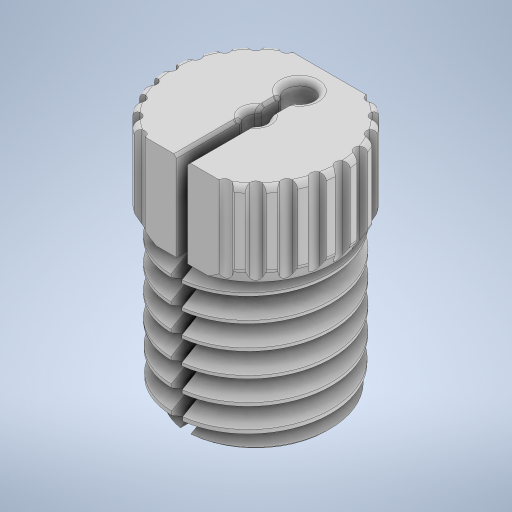
# Autodesk Inventor part: Ferula FOV5
Saved by Autodesk Inventor 2024.2 (Build 282272000, 272)
## iProperties
Created: 2025-08-06
Part Number: Ferula FOV5
Material: Generic
Document SubType Name: Modeling
Designer: ja.restrepo1
Density: 1 g/cm^3
Appearance: Default
Author: ja.restrepo1
Autodesk Inventor part; units mm, degrees
ref_plane "YZ Plane" through (0, 0, 0) normal (1, 0, 0) x (0, 1, 0)
ref_plane "XZ Plane" through (0, 0, 0) normal (0, 1, 0) x (-1, 0, 0)
ref_plane "XY Plane" through (0, 0, 0) normal (0, 0, 1) x (1, 0, 0)
sketch "Sketch1" plane through (0, 0, 0) normal (1, 0, 0) x (0, 0, -1)
  line L0 (-0.725, 5.6) -> (-0.725, 10.6)
  line L1 (-0.725, 10.6) -> (-5.825, 10.6)
  line L2 (-2.7455, -0.9529) -> (-2.1722, 5.6)
  line L3 (-2.1722, 5.6) -> (-0.725, 5.6)
  line L4 (-5.825, 3.6) -> (-5.756, -0.353)
  line L5 (-5.1455, -0.9529) -> (-2.7455, -0.9529)
  line L6 (-5.825, 10.6) -> (-5.825, 3.6)
  line L7 (0, -3.2635) -> (0, 12.9106) projected
  line L8 (-5.1455, -0.9529) -> (-5.756, -0.353)
  point P0 (0, 0)
  point P1 (-5.7455, -0.9529)
  point P2 (0, 0)
  dimension "d1" = 5
  dimension "d4" = 3
  dimension "d8" = 7
  dimension "d11" = 0.725
  dimension "d12" = 5.1
  dimension "d13" = 179
  dimension "d41" = 5.825
  dimension "d65" = 0.6
  dimension "d66" = 0.6
  dimension "d67" = 11.5529
  dimension "d98" = 5.6
  dimension "d100" = 95
  dimension "d111" = 1.4472
  constraints: 17 end point, 2 coincident, 2 perpendicular, 2 point on line, 1 horizontal, 1 parallel, 1 vertical
  measures "d1" distance of L3.end L0.end
  measures "d4" distance of point (-5.746, -0.953) L5.end
  measures "d8" distance of L6.start L4.start
  measures "d11" distance from line of point (0, 0) L0
  measures "d12" distance between parallel lines of L0 L6
  measures "d13" angle of L4 L6
  measures "d41" distance between parallel lines of L6 L7
  measures "d65" distance of L5.start point (-5.746, -0.953)
  measures "d66" distance of L4.end point (-5.746, -0.953)
  measures "d67" distance between parallel lines of L5 L1
  measures "d98" distance from line of L3 point (0, 0)
  measures "d100" angle of L5 L2
  measures "d111" distance of L2.end L3.end
revolve "Ferula Optica" add sketch "Sketch1" angle 360 about axis through (0, -10, 0) along (0, 1, 0)
fillet "Fillet1" radius 0.2 1 edges at (0, -0.9529, -2.7455)
fillet "Fillet2" radius 0.4 1 edges at (0, 10.6, -5.825)
chamfer "Chamfer1" distance 0.6 angle 45 1 edges at (0, 5.6, -2.1722)
sketch "Sketch5" plane through (0, 0, 0) normal (0, 0, 1) x (1, 0, 0)
  line L0 (0, -1) -> (-4.5, -1) construction
  line L1 (-4.5, -1) -> (-5.8856, -1.8)
  line L2 (-5.8856, -1.8) -> (-5.8856, -0.2)
  line L3 (-5.8856, -0.2) -> (-4.5, -1)
  point P0 (0, 0)
  point P1 (-5.4238, -1)
  dimension "d42" = 4.5
  dimension "d43" = 1
  dimension "d44" = 1.6
  constraints: 8 end point, 1 horizontal, 1 vertical, 1 vertical alignment, 7 other
  measures "d42" distance of L0.start L0.end
  measures "d43" distance from line of point (0, 0) L0
  measures "d44" distance of L1.end L2.end
coil "M12 (5.71)" sketch "Sketch5" operation cut axis through (0, -10, 0) along (0, 1, 0) pitch 1.75 turns 7 hand right
sketch "Sketch7" plane through (0, 0, 0) normal (0, 0, 1) x (1, 0, 0)
  line L0 (-0.725, 16.5) -> (-0.725, 10)
  line L1 (-0.725, 10) -> (-5.725, 10)
  line L2 (-5.725, 10) -> (-5.725, 10.4)
  line L3 (-6.325, 11) -> (-6.4, 11)
  line L4 (-6.4, 11) -> (-6.4, 16.5)
  line L5 (-6.4, 16.5) -> (-0.725, 16.5)
  line L6 (2.2245, 5.0023) -> (1.5722, 5.6) projected
  line L7 (1.5722, 5.6) -> (0.725, 5.6) projected
  line L8 (0.725, 5.6) -> (0.725, 10.6) projected
  line L9 (0.725, 10.6) -> (4.8897, 10.6) projected
  line L10 (5.1455, -0.9529) -> (2.9288, -0.9529) projected
  arc A0 (2.7296, -0.7703) -> (2.9288, -0.9529) centre (2.9288, -0.7529) ccw projected
  line L11 (2.7296, -0.7703) -> (2.2245, 5.0023) projected
  line L12 (-1.5722, 5.6) -> (-2.2245, 5.0023) projected
  line L13 (-2.2245, 5.0023) -> (-2.7296, -0.7703) projected
  arc A1 (-2.9288, -0.9529) -> (-2.7296, -0.7703) centre (-2.9288, -0.7529) ccw projected
  line L14 (-2.9288, -0.9529) -> (-4.5816, -0.9529) projected
  line L15 (5.4373, -0.6662) -> (5.1455, -0.9529) projected
  line L16 (-5.425, 10.6) -> (-0.725, 10.6) projected
  line L17 (-0.725, 10.6) -> (-0.725, 5.6) projected
  line L18 (-0.725, 5.6) -> (-1.5722, 5.6) projected
  line L19 (0, -3.3465) -> (0, 19.8077) projected
  line L20 (5.8079, 2.6199) -> (5.8037, 2.3777) projected
  line L21 (5.7777, 0.8873) -> (5.7728, 0.6099) projected
  line L22 (-5.8191, 3.2616) -> (-5.823, 3.4862) projected
  line L23 (5.825, 9.61) -> (5.825, 9.39) projected
  line L24 (5.825, 7.86) -> (5.825, 7.64) projected
  line L25 (5.825, 6.11) -> (5.825, 5.89) projected
  line L26 (5.825, 4.36) -> (5.825, 4.14) projected
  line L27 (-5.7882, 1.4938) -> (-5.7928, 1.7536) projected
  line L28 (-5.825, 8.515) -> (-5.825, 8.735) projected
  line L29 (-5.825, 6.765) -> (-5.825, 6.985) projected
  line L30 (-5.825, 5.015) -> (-5.825, 5.235) projected
  arc A2 (-5.425, 10.6) -> (-5.8201, 10.2622) centre (-5.425, 10.2) ccw projected
  line L31 (-6.325, 11) -> (-5.725, 10)
  line L32 (-5.7574, -0.2741) -> (-4.5816, -0.9529) projected
  line L33 (-5.756, -0.353) -> (-5.7574, -0.2741) projected
  line L34 (-5.1455, -0.9529) -> (-5.756, -0.353) projected
  line L35 (-4.5816, -0.9529) -> (-5.1455, -0.9529) projected
  line L36 (-5.7574, -0.2741) -> (-5.7625, 0.0211) projected
  point P0 (0, 0)
  point P1 (-5.7018, 10.2805)
  point P2 (-5.366, 10)
  point P3 (-0.725, 10.6)
  point P4 (-0.725, 10)
  point P5 (-6.4, 11)
  dimension "d69" = 6.5
  dimension "d70" = 6.4
  dimension "d71" = 5
  dimension "d73" = 10
  dimension "d76" = 1
  dimension "d112" = 149.036
  constraints: 14 end point, 5 perpendicular, 1 collinear, 1 vertical, 26 other
  measures "d69" distance of L0.start L0.end
  measures "d70" distance from line of L4 point (0, 0)
  measures "d71" distance of L0.end L1.end
  measures "d73" distance from line of L1 point (0, 0)
  measures "d76" distance between parallel lines of L3 L1
  measures "d112" angle of L4 L31
revolve "cabeza" add sketch "Sketch7" angle 360 about axis through (0, -10, 0) along (0, 1, 0) contours L0 L1 L31 L3 L4 L5
fillet "Fillet4" radius 0.4 2 edges at (6.4, 16.5, 0) (6.4, 11, 0)
sketch "Sketch9" plane through (0, 16.5, 0) normal (0, 1, 0) x (1, 0, 0)
  line L0 (-0.3464, 6.034) -> (-0.75, 6.733)
  line L1 (-0.75, 6.733) -> (0.75, 6.733)
  line L2 (0.75, 6.733) -> (0.3464, 6.034)
  arc A0 (-0.3464, 6.034) -> (0.3464, 6.034) centre (0, 6.234) ccw
  point P0 (0, 0)
  point P1 (0, 6.3)
  point P2 (0, 5.434)
  dimension "d78" = 1.5
  dimension "d79" = 6.3
  dimension "d85" = 0.4
  constraints: 6 end point, 2 point on circle, 2 point on line, 2 tangent, 1 centre point, 1 horizontal, 1 vertical alignment, 7 other
  measures "d78" distance of L0.end L1.end
  measures "d79" distance of point (0, 6.3) point (0, 0)
  measures "d85" radius of A0
extrude "antidezlis" cut sketch "Sketch9" against normal blind 6.5
pattern_circular "Circular Pattern2" count 24 over 360 about axis through (0, 16.1, 0) along (0, 1, 0) of "antidezlis"
sketch "Sketch10" plane through (0, 16.5, -6.234) normal (0, 1, 0) x (1, 0, 0)
  arc A0 (0.4, -3.9505) -> (-0.4, -3.9505) centre (0, -3.034) ccw
  line L0 (-0.4, -3.9505) -> (-0.4, -12.9505)
  line L1 (-0.4, -12.9505) -> (0.4, -12.9505)
  line L2 (0.4, -12.9505) -> (0.4, -3.9505)
  point P0 (0, -6.234)
  point P1 (0, -12.9505)
  dimension "d86" = 2
  dimension "d88" = 3.2
  dimension "d113" = 9
  dimension "d114" = 0.8
  constraints: 8 end point, 2 coincident, 2 point on circle, 2 vertical alignment, 1 centre point, 1 midpoint, 1 parallel, 1 perpendicular, 1 vertical
  measures "d86" diameter of A0
  measures "d88" distance of A0.centre point (0, -6.234)
  measures "d113" distance from line of L1 L0.start
  measures "d114" distance of L1.end L0.end
extrude "ranura" cut sketch "Sketch10" against normal through all
fillet "Fillet5" radius 0.4 5 edges at (0, 16.5, -4.2) (-0.725, 16.5, 0) (0.725, 16.5, 0) (-0.725, 5.6, 0) (0.725, 5.6, 0)
sketch "Sketch11" plane through (0, 16.5, -6.234) normal (0, 1, 0) x (1, 0, 0)
  line L0 (-5, 0.666) -> (-5, -0.834)
  line L1 (-5, -11.634) -> (-5, -13.134)
  line L2 (5, -11.634) -> (5, -13.134)
  line L3 (5, 0.666) -> (5, -0.834)
  line L4 (-5, 0.666) -> (5, 0.666)
  line L5 (-5, -0.834) -> (5, -0.834)
  line L6 (5, -13.134) -> (-5, -13.134)
  line L7 (5, -11.634) -> (-5, -11.634)
  line L8 (0, -0.834) -> (0, -11.634) construction
  point P0 (0, -6.234)
  point P1 (0, -6.234)
  dimension "d119" = 10.8
  dimension "d120" = 1.5
  dimension "d121" = 10
  constraints: 18 end point, 4 point on line, 3 midpoint, 2 parallel, 2 perpendicular, 2 vertical alignment, 1 coincident, 1 collinear, 1 horizontal
  measures "d119" distance of L8.start L8.end
  measures "d120" distance of L0.start L0.end
  measures "d121" distance of L0.start L3.start
extrude "caja 10mm" cut sketch "Sketch11" against normal blind 6.7 contours L7 L2 L6 L1
chamfer "Chamfer3" distance 0.2 angle 45 12 edges at (-0.4, 16.5, 3.2257) (-0.4, 16.5, -1.4549) (-0.4, 16.3842, 0.7426) (-0.4, 11.05, 0.6047) (-0.4, 5.7158, 0.7426) (-0.4, 5.6, 1.286) (0.4, 16.5, -1.4549) (0.4, 16.5, 3.2257) (0.4, 16.3842, 0.7426) (0.4, 11.05, 0.6047) (0.4, 5.7158, 0.7426) (0.4, 5.6, 1.286)
extrude "Extrusion8" cut sketch "Sketch11" against normal blind 7.2 contours L4 L3 L5 L0
equation "\"d66\" = d65"
body "Solid1"
